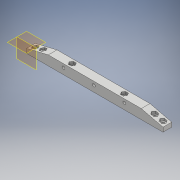
# Autodesk Inventor part: new_wheel_support_v2
Saved by Autodesk Inventor 2017 (Build 210142000, 142)
## iProperties
Created: 2017-08-21
Part Number: new_wheel_support_v2
Material: Generic
Document SubType Name: Modeling
Designer: ndz
Density: 1 g/cm^3
Appearance: Default
Author: ndz
Autodesk Inventor part; units mm, degrees
ref_plane "YZ Plane" through (0, 0, 0) normal (1, 0, 0) x (0, 1, 0)
ref_plane "XZ Plane" through (0, 0, 0) normal (0, 1, 0) x (-1, 0, 0)
ref_plane "XY Plane" through (0, 0, 0) normal (0, 0, 1) x (1, 0, 0)
sketch "Sketch1" plane through (0, 0, 0) normal (0, 0, 1) x (1, 0, 0)
  line L0 (0, 0) -> (157, 0)
  line L1 (157, 0) -> (157, 10)
  line L2 (157, 10) -> (0, 10)
  line L3 (0, 10) -> (0, 0)
  circle A0 centre (47.5, 5) radius 1.6
  circle A1 centre (107.5, 5) radius 1.6
  circle A2 centre (152, 5) radius 1.6
  circle A3 centre (142.5, 5) radius 1.6
  circle A4 centre (5, 5) radius 1.6
  circle A5 centre (14, 5) radius 1.6
  dimension "d1" = 10
  dimension "d2" = 90
  dimension "d4" = 3.2
  dimension "d6" = 3.2
  dimension "d7" = 3.2
  dimension "d8" = 60
  dimension "d9" = 44.5
  dimension "d26" = 3.2
  dimension "d27" = 35
  dimension "d28" = 3.2
  dimension "d29" = 42.5
  dimension "d32" = 5
  dimension "d33" = 5
  dimension "d34" = 3.2
  dimension "d35" = 9
  constraints: 8 end point, 6 centre point, 2 perpendicular, 1 horizontal
  measures "d1" distance of L0.end L1.end
  measures "d2" angle of L1 L0
  measures "d4" diameter of A0
  measures "d6" diameter of A1
  measures "d7" diameter of A2
  measures "d8" distance of A1.centre A0.centre
  measures "d9" distance of A2.centre A1.centre
  measures "d26" diameter of A3
  measures "d27" distance of A3.centre A1.centre
  measures "d28" diameter of A4
  measures "d29" distance of A4.centre A0.centre
  measures "d32" distance from line of L3 A4.centre
  measures "d33" distance from line of L1 A2.centre
  measures "d34" diameter of A5
  measures "d35" distance of A5.centre A4.centre
ref_plane "Work Plane2" through (0, 0, 0) normal (0, -1, 0) x (1, 0, 0)
sketch "Sketch2" plane through (0, 0, 0) normal (0, -1, 0) x (1, 0, 0)
  circle A0 centre (42.5, 7) radius 1.6
  circle A1 centre (112.5, 7) radius 1.6
  circle A2 centre (77.5, 7) radius 1.6
  dimension "d13" = 3.2
  dimension "d15" = 3.2
  dimension "d16" = 70
  dimension "d17" = 3.2
  dimension "d18" = 35
  constraints: 3 centre point
  measures "d13" diameter of A0
  measures "d15" diameter of A1
  measures "d16" distance of A0.centre A1.centre
  measures "d17" diameter of A2
  measures "d18" distance of A0.centre A2.centre
ref_plane "Work Plane1" through (0, 0, 11) normal (0, 0, 1) x (1, 0, 0)
extrude "Extrusion4" add sketch "Sketch1" along normal blind 11
extrude "Extrusion5" cut sketch "Sketch2" against normal up to next
sketch "Sketch7" plane through (0, 0, 0) normal (0, -1, 0) x (1, 0, 0)
  line L0 (0, 11) -> (0, 5)
  line L1 (0, 11) -> (25, 11)
  line L2 (25, 11) -> (0, 5)
  point P0 (0, 0)
  constraints: 6 end point
extrude "Extrusion6" cut sketch "Sketch7" against normal up to next
sketch "Sketch8" plane through (0, 0, 0) normal (0, -1, 0) x (1, 0, 0)
  line L0 (157, 11) -> (25, 11) projected
  line L1 (157, 11) -> (157, 5)
  line L2 (157, 0) -> (157, 11) projected
  line L3 (157, 0) -> (157, 11) projected
  line L4 (157, 11) -> (132, 11)
  line L5 (25, 11) -> (157, 11) projected
  line L6 (132, 11) -> (157, 5)
  point P0 (0, 0)
  constraints: 6 end point, 2 point on line
extrude "Extrusion7" cut sketch "Sketch8" against normal up to next
sketch "Sketch5" plane through (0, 0, 11) normal (0, 0, 1) x (1, 0, 0)
  circle A0 centre (47.5, 5) radius 1.6 projected
  line L0 (50.9064, 5) -> (49.2032, 2.05)
  line L1 (49.2032, 2.05) -> (45.7968, 2.05)
  line L2 (45.7968, 2.05) -> (44.0936, 5)
  line L3 (44.0936, 5) -> (45.7968, 7.95)
  line L4 (45.7968, 7.95) -> (49.2032, 7.95)
  line L5 (49.2032, 7.95) -> (50.9064, 5)
  circle A1 centre (107.5, 5) radius 1.6 projected
  line L6 (110.9064, 5) -> (109.2032, 2.05)
  line L7 (109.2032, 2.05) -> (105.7968, 2.05)
  line L8 (105.7968, 2.05) -> (104.0936, 5)
  line L9 (104.0936, 5) -> (105.7968, 7.95)
  line L10 (105.7968, 7.95) -> (109.2032, 7.95)
  line L11 (109.2032, 7.95) -> (110.9064, 5)
  dimension "d44" = 5.9
  dimension "d45" = 5.9
  constraints: 24 end point, 2 coincident, 26 other
  measures "d44" distance between parallel lines of L7 L10
  measures "d45" distance between parallel lines of L1 L4
sketch "Sketch9" plane through (0, 0, 11) normal (0, 0, 1) x (1, 0, 0)
  circle A0 centre (14, 5) radius 1.6 projected
  line L0 (17.4064, 5) -> (15.7032, 2.05)
  line L1 (15.7032, 2.05) -> (12.2968, 2.05)
  line L2 (12.2968, 2.05) -> (10.5936, 5)
  line L3 (10.5936, 5) -> (12.2968, 7.95)
  line L4 (12.2968, 7.95) -> (15.7032, 7.95)
  line L5 (15.7032, 7.95) -> (17.4064, 5)
  circle A1 centre (142.5, 5) radius 1.6 projected
  line L6 (145.9064, 5) -> (144.2032, 2.05)
  line L7 (144.2032, 2.05) -> (140.7968, 2.05)
  line L8 (140.7968, 2.05) -> (139.0936, 5)
  line L9 (139.0936, 5) -> (140.7968, 7.95)
  line L10 (140.7968, 7.95) -> (144.2032, 7.95)
  line L11 (144.2032, 7.95) -> (145.9064, 5)
  point P0 (0, 0)
  dimension "d51" = 5.9
  dimension "d52" = 5.9
  constraints: 24 end point, 2 coincident, 26 other
  measures "d51" distance between parallel lines of L7 L10
  measures "d52" distance between parallel lines of L1 L4
sketch "Sketch10" plane through (0, 0, 11) normal (0, 0, 1) x (1, 0, 0)
  line L0 (8.4064, 5) -> (6.7032, 2.05)
  line L1 (6.7032, 2.05) -> (3.2968, 2.05)
  line L2 (3.2968, 2.05) -> (1.5936, 5)
  line L3 (1.5936, 5) -> (3.2968, 7.95)
  line L4 (3.2968, 7.95) -> (6.7032, 7.95)
  line L5 (6.7032, 7.95) -> (8.4064, 5)
  line L6 (155.4064, 5) -> (153.7032, 2.05)
  line L7 (153.7032, 2.05) -> (150.2968, 2.05)
  line L8 (150.2968, 2.05) -> (148.5936, 5)
  line L9 (148.5936, 5) -> (150.2968, 7.95)
  line L10 (150.2968, 7.95) -> (153.7032, 7.95)
  line L11 (153.7032, 7.95) -> (155.4064, 5)
  point P0 (0, 0)
  point P1 (5, 5)
  point P2 (152, 5)
  dimension "d53" = 5.9
  dimension "d54" = 5.9
  constraints: 24 end point, 26 other
  measures "d53" distance between parallel lines of L7 L10
  measures "d54" distance between parallel lines of L1 L4
extrude "Extrusion8" cut sketch "Sketch5" against normal blind 3
extrude "Extrusion9" cut sketch "Sketch9" against normal blind 5
extrude "Extrusion10" cut sketch "Sketch10" against normal blind 7
body "Solid1"
